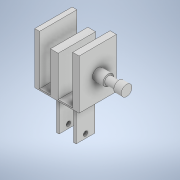
# Autodesk Inventor part: grip - Copy1-1
Saved by Autodesk Inventor 2021 (Build 250183000, 183)
## iProperties
Created: 2021-05-09
Part Number: grip - Copy1-1
Material: Generic
Document SubType Name: Modeling
Designer: Alsayaary
Density: 1 g/cm^3
Appearance: Default
Author: Abdulrahman
Autodesk Inventor part; units mm, degrees
ref_plane "YZ Plane" through (0, 0, 0) normal (1, 0, 0) x (0, 1, 0)
ref_plane "XZ Plane" through (0, 0, 0) normal (0, 1, 0) x (-1, 0, 0)
ref_plane "XY Plane" through (0, 0, 0) normal (0, 0, 1) x (1, 0, 0)
sketch "Sketch1" plane through (0, 0, 0) normal (0, 0, 1) x (1, 0, 0)
  line L0 (-38, 45.376) -> (-29, 45.376)
  line L1 (-29, 45.376) -> (-29, 48)
  line L2 (-29, 141) -> (-29, 48)
  line L3 (-38, 141) -> (-29, 141)
  line L4 (-38, 45.376) -> (-38, 141)
  line L5 (0, 45.376) -> (45, 45.376)
  line L6 (45, 138) -> (45, 45.376)
  line L7 (33, 138) -> (45, 138)
  line L8 (33, 48) -> (33, 138)
  line L9 (6, 48) -> (33, 48)
  line L10 (6, 48) -> (6, 123)
  line L11 (6, 123) -> (-8.5, 123)
  line L12 (-8.5, 123) -> (-8.5, 48)
  line L13 (0, 48) -> (-8.5, 48)
  line L14 (0, 45.376) -> (0, 48)
  line L15 (0, 48) -> (0, 45.376)
  line L16 (-29, 48) -> (0, 48)
  line L17 (-29, 45.376) -> (-29, 48)
  line L18 (0, 45.376) -> (-29, 45.376)
  point P0 (0, 0)
  point P1 (276, 309.9765)
  dimension "GRIP3_W" = 12
  dimension "GRIP3_MID_THICK" = 14.5
  dimension "GRIP3_LEFT_THICK" = 9
  dimension "GRIP3_H" = 92.624
  dimension "GRIP3_MIDDLE_H" = 75
  dimension "GRIP3_LEFT_H" = 95.624
  dimension "GRIP3_W_ALL" = 83
  dimension "GRIP3_T" = 2.624
  dimension "GRIP3_T_2" = 2.624
  constraints: 38 end point
  measures "GRIP3_W" distance of L7.start L6.start
  measures "GRIP3_MID_THICK" distance of L10.end L11.end
  measures "GRIP3_LEFT_THICK" distance of L3.start L2.start
  measures "GRIP3_H" distance of L6.start L5.end
  measures "GRIP3_MIDDLE_H" distance of L9.start L10.end
  measures "GRIP3_LEFT_H" distance of L0.start L3.start
  measures "GRIP3_W_ALL" distance between parallel lines of L6 L4
  measures "GRIP3_T" distance between parallel lines of L5 L9
  measures "GRIP3_T_2" distance between parallel lines of L18 L16
extrude "Extrusion1" add sketch "Sketch1" along normal mid plane 70
sketch "Sketch2" plane through (0, 0, 0) normal (0, 0, 1) x (1, 0, 0)
  line L0 (-29, 45.376) -> (45, 45.376) projected
  line L1 (-15, 45.376) -> (-10, 45.376)
  line L2 (-10, 45.376) -> (-10, -24.624)
  line L3 (-10, -24.624) -> (-15, -24.624)
  line L4 (-15, -24.624) -> (-15, 45.376)
  line L5 (17, 45.376) -> (22, 45.376)
  line L6 (22, 45.376) -> (22, -24.624)
  line L7 (22, -24.624) -> (17, -24.624)
  line L8 (17, -24.624) -> (17, 45.376)
  line L9 (45, 45.376) -> (45, 138) projected
  line L10 (-38, 141) -> (-38, 45.376) projected
  point P0 (0, 0)
  point P1 (-10, 45.376)
  point P2 (22, 45.376)
  dimension "GRIP3_MTG" = 70
  dimension "GRIP3_MTG_TH" = 5
  dimension "GRIP3_LOC" = 23
  dimension "d16" = 23
  constraints: 16 end point, 4 parallel, 3 point on line, 2 horizontal, 2 perpendicular, 1 collinear
  measures "GRIP3_MTG" distance of L3.end L1.start
  measures "GRIP3_MTG_TH" distance of L2.end L3.end
  measures "GRIP3_LOC" distance between parallel lines of L9 L6
  measures "d16" distance between parallel lines of L10 L4
extrude "Extrusion2" add sketch "Sketch2" along normal mid plane 35
sketch "Sketch3" plane through (0, 0, 0) normal (1, 0, 0) x (0, 1, 0)
  circle A0 centre (-16.624, 0) radius 4.123
  line L0 (-24.624, -17.5) -> (-24.624, 17.5) projected
  line L1 (45.376, -17.5) -> (-24.624, -17.5) projected
  point P0 (0, 0)
  dimension "PIN_HOLE_DIAM" = 8.246
  dimension "LOC_PIN_HOLE" = 8
  dimension "LOC_HOLE" = 17.5
  constraints: 1 centre point
  measures "PIN_HOLE_DIAM" diameter of A0
  measures "LOC_PIN_HOLE" distance from line of L0 A0.centre
  measures "LOC_HOLE" distance from line of L1 A0.centre
extrude "Extrusion3" cut sketch "Sketch3" along normal blind 35 and the other way blind 35
sketch "Sketch4" plane through (45, 45.376, 35) normal (1, 0, 0) x (0, 0, -1)
  circle A0 centre (35, 46.312) radius 10
  line L0 (70, 92.624) -> (70, 0) projected
  line L1 (70, 0) -> (0, 0) projected
  point P0 (35, -45.376)
  dimension "PIN_DIAM1" = 20
  dimension "LOC_PIN" = 35
  dimension "d26" = 46.312
  constraints: 1 centre point
  measures "PIN_DIAM1" diameter of A0
  measures "LOC_PIN" distance from line of L0 A0.centre
  measures "d26" distance from line of L1 A0.centre
extrude "Extrusion4" add sketch "Sketch4" along normal blind 19.946
sketch "Sketch5" plane through (64.946, 91.688, 0) normal (1, 0, 0) x (0, 0, -1)
  circle A0 centre (0, 0) radius 7
  point P0 (0, -91.688)
  dimension "PIN_DIAME2" = 14
  constraints: 1 centre point
  measures "PIN_DIAME2" diameter of A0
extrude "Extrusion5" add sketch "Sketch5" along normal blind 20
sketch "Sketch6" plane through (84.946, 91.688, 0) normal (1, 0, 0) x (0, 0, -1)
  circle A0 centre (0, 0) radius 10
  point P0 (0, -91.688)
  dimension "PIN_DIAM3" = 20
  constraints: 1 centre point
  measures "PIN_DIAM3" diameter of A0
extrude "Extrusion6" add sketch "Sketch6" along normal blind 14
equation "\"GRIP3_T_2\" = GRIP3_T"
equation "\"d16\" = GRIP3_LOC"
equation "\"LOC_HOLE\" = 0.5 * GRIP3_MTG_EXTR"
equation "\"LOC_PIN\" = 0.5 * GRIP3_EXTR"
equation "\"d26\" = 0.5 * GRIP3_H"
equation "\"PIN_DIAM3\" = PIN_DIAM1"
equation "\"PIN3_H\" = PIN_DIAME2"
equation "\"GRIP3_MTG_EXTR\" = 35"
equation "\"GRIP3_EXTR\" = 70"
body "Solid1"
